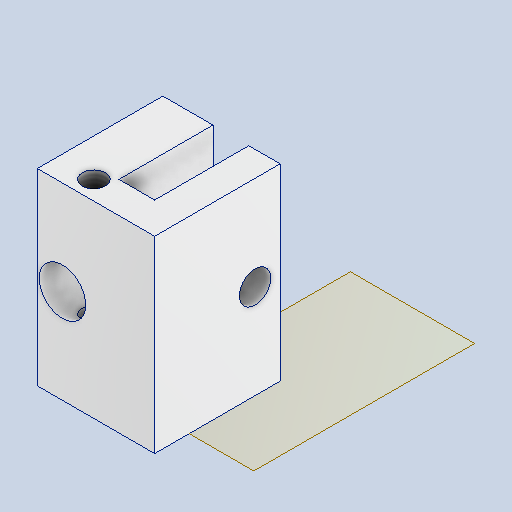
# Autodesk Inventor part: Katze_Lagerhalter_hinten
Saved by Autodesk Inventor 2025 (Build 290162010, 162A)
## iProperties
Created: 2024-11-11
Part Number: Katze_Lagerhalter_hinten
Material: Aluminium 6061(1)
Document SubType Name: Modeling
Designer: Admin
Density: 2.7 g/cm^3
Appearance: Aluminium - flach(1)
Author: Admin
Autodesk Inventor part; units mm, degrees
ref_plane "YZ Plane" through (0, 0, 0) normal (1, 0, 0) x (0, 1, 0)
ref_plane "XZ Plane" through (0, 0, 0) normal (0, 1, 0) x (-1, 0, 0)
ref_plane "XY Plane" through (0, 0, 0) normal (0, 0, 1) x (1, 0, 0)
ref_plane "Arbeitsebene1" through (0, 0, 0) normal (0, 0, 1) x (1, 0, 0)
sketch "Skizze1" plane through (0, 0, 0) normal (0, 0, 1) x (1, 0, 0)
  line L0 (-0.4, -3.1) -> (-5.4, -3.1)
  line L1 (-11.1, -3.1) -> (-19.1, -3.1)
  line L2 (-5.4, -3.1) -> (-5.4, -18.1)
  line L3 (-5.4, -18.1) -> (-11.1, -18.1)
  line L4 (-0.4, -23.1) -> (-0.4, -3.1)
  line L5 (-19.1, -23.1) -> (-0.4, -23.1)
  line L6 (-19.1, -3.1) -> (-19.1, -23.1)
  line L7 (-11.1, -18.1) -> (-11.1, -3.1)
  line L8 (-9, -16) -> (-9, -18.1) construction
  line L9 (-9, -16) -> (-11.1, -16) construction
  line L10 (-7.5, -16) -> (-5.4, -16) construction
  line L11 (-7.5, 1) -> (7.5, 1) projected
  line L12 (7.5, 1) -> (7.5, 16) projected
  line L13 (7.5, 16) -> (9, 16) projected
  line L14 (9, 16) -> (9, -16) projected
  line L15 (9, -16) -> (7.5, -16) projected
  line L16 (7.5, -16) -> (7.5, -1) projected
  line L17 (7.5, -1) -> (-7.5, -1) projected
  line L18 (-7.5, -1) -> (-7.5, -16) projected
  line L19 (-7.5, -16) -> (-9, -16) projected
  line L20 (-9, -16) -> (-9, 16) projected
  line L21 (-9, 16) -> (-7.5, 16) projected
  line L22 (-7.5, 16) -> (-7.5, 1) projected
  point P0 (0, 0)
  dimension "d0" = 5
  dimension "d1" = 8
  dimension "d2" = 5
  dimension "d3" = 20
  dimension "d4" = 2.1
  constraints: 22 end point, 10 perpendicular, 3 equal length, 3 point on line, 1 horizontal
  measures "d0" distance between parallel lines of L5 L3
  measures "d1" distance between parallel lines of L7 L6
  measures "d2" distance between parallel lines of L2 L4
  measures "d3" distance between parallel lines of L5 L1
  measures "d4" distance of L9.start L9.end
extrude "Extrusion1" add sketch "Skizze1" along normal blind 30 contours L4 L5 L6 L1 L7 L3 L2 L0
sketch "Skizze3" plane through (-5.4, -18.1, 0) normal (-1, 0, 0) x (0, 0, 1)
  line L0 (15, 6) -> (15, 15) construction
  line L1 (15, 6) -> (0, 6) construction
  line L2 (30, 15) -> (30, 0) construction
  line L3 (0, 15) -> (30, 15) construction
  line L4 (0, 15) -> (0, 0) construction
  line L5 (15, 6) -> (30, 6) construction
  point P0 (0, 18.1)
  dimension "d74" = 9
  constraints: 6 end point, 3 perpendicular, 2 point on line, 1 coincident, 1 collinear, 1 midpoint
  measures "d74" distance of L0.start L0.end
hole "GLHU" at (-5.4, -12.1, 15) direction (1, 0, 0) diameter 1.567 depth 4 tip angle 118 thread size "M2x0.4" class "6H" standard "ISO Metric profile"
sketch "Skizze9" plane through (-11.1, -18.1, 0) normal (0, 1, 0) x (1, 0, 0)
  line L0 (5.7, 0) -> (0, 0) construction
  line L1 (0, 0) -> (0, -30) construction
  line L2 (5.7, -30) -> (0, -30) construction
  line L3 (5.7, 0) -> (5.7, -30) construction
  line L4 (2.85, -30) -> (2.85, -15) construction
  line L5 (2.85, -15) -> (0, -15) construction
  line L6 (2.85, -15) -> (2.85, 0) construction
  point P0 (11.1, 0)
  constraints: 6 end point, 3 midpoint, 1 coincident, 1 collinear, 1 vertical
hole "GLHH" at (-8.25, -18.1, 15) direction (0, -1, 0) diameter 1.567 depth 4 tip angle 118 thread size "M2x0.4" class "6H" standard "ANSI Metric M Profile"
sketch "Skizze10" plane through (-11.1, -18.1, 0) normal (1, 0, 0) x (0, 0, -1)
  line L0 (-30, 0) -> (-30, 15) construction
  line L1 (0, 15) -> (-30, 15) construction
  line L2 (0, 0) -> (0, 15) construction
  line L3 (-30, 11) -> (-15, 11) construction
  line L4 (-15, 11) -> (0, 11) construction
  point P0 (0, 18.1)
  dimension "d75" = 4
  constraints: 4 end point, 3 point on line, 1 coincident, 1 collinear, 1 horizontal
  measures "d75" distance from line of L1 L3.end
hole "GLHO" at (-11.1, -7.1, 15) direction (-1, 0, 0) diameter 1.567 depth 4 tip angle 118 thread size "M2x0.4" class "6H" standard "ANSI Metric M Profile"
sketch "Skizze11" plane through (-11.1, -18.1, 0) normal (1, 0, 0) x (0, 0, -1)
  circle A0 centre (-15, 6) radius 0.7835 construction
  line L0 (0, 15) -> (0, 0) construction
  line L1 (0, 0) -> (-30, 0) construction
  line L2 (-30, 15) -> (-30, 0) construction
  line L3 (0, 15) -> (-30, 15) construction
  point P0 (0, 18.1)
  constraints: 1 coincident
hole "DLHO" at (-11.1, -12.1, 15) direction (-1, 0, 0) diameter 5 end through all
sketch "Skizze12" plane through (-5.4, -18.1, 0) normal (-1, 0, 0) x (0, 0, 1)
  circle A0 centre (15, 11) radius 0.7835 construction
  point P0 (0, 18.1)
  constraints: 1 coincident
hole "DLHU" at (-5.4, -7.1, 15) direction (1, 0, 0) diameter 5 end through all
sketch "Skizze6" plane through (-19.1, -3.1, 0) normal (0, 1, 0) x (1, 0, 0)
  line L0 (8, 0) -> (0, 0) projected
  line L1 (0, 0) -> (0, -30) projected
  line L2 (8, -30) -> (0, -30) projected
  line L3 (8, 0) -> (8, -30) projected
  line L4 (5.5, -30) -> (5.5, -27) construction
  line L5 (5.5, -27) -> (5.5, -3) construction
  line L6 (5.5, -3) -> (5.5, 0) construction
  line L7 (5.5, -3) -> (8, -3) construction
  point P0 (19.1, 0)
  dimension "d42" = 2.5
  dimension "d43" = 3
  constraints: 8 end point, 5 point on line, 2 coincident, 1 collinear, 1 perpendicular, 1 vertical
  measures "d42" distance of L5.end L7.end
  measures "d43" distance of L5.end L6.end
hole "Zentrierbolzen" at (-13.6, -3.1, 3) at (-13.6, -3.1, 27) direction (0, -1, 0) diameter 2 depth 5 tip angle 118
sketch "Skizze8" plane through (-19.1, -23.1, 0) normal (0, -1, 0) x (1, 0, 0)
  line L0 (0, 0) -> (18.7, 0) construction
  line L1 (18.7, 0) -> (18.7, 30) construction
  line L2 (0, 30) -> (18.7, 30) construction
  line L3 (0, 0) -> (0, 30) construction
  line L4 (4, 0) -> (4, 15) construction
  line L5 (4, 15) -> (4, 30) construction
  point P0 (19.1, 0)
  point P1 (0, 15)
  dimension "d58" = 4
  constraints: 4 end point, 3 point on line, 1 coincident, 1 collinear, 1 midpoint, 1 vertical
  measures "d58" distance of point (0, 15) L4.end
hole "LK-Verschraubung" at (-15.1, -23.1, 15) direction (0, 1, 0) diameter 4 end through all counterbore diameter 7.4 counterbore depth 14
sketch "Skizze13" plane through (0, 0, 0) normal (0, 0, -1) x (-1, 0, 0)
  line L0 (11.4, -9.1) -> (11.4, -23.1) construction
  line L1 (5.4, -18.1) -> (11.1, -18.1) construction
  line L2 (13.1, -20.1) -> (19.1, -20.1) construction
  line L3 (19.1, -3.1) -> (19.1, -23.1) construction
  line L4 (19.1, -23.1) -> (19.1, -20.1) construction
  point P0 (0, 0)
  dimension "d109" = 6
  dimension "d110" = 3
  constraints: 4 end point, 1 collinear, 1 horizontal, 1 point on line
  measures "d109" distance of L2.start L2.end
  measures "d110" distance of L3.end L2.end
hole "seiloese" at (-13.1, -20.1, 0) direction (0, 0, 1) diameter 3.6881 end through all thread size "M4.5x0.75" class "6H" standard "ANSI Metric M Profile"
thread "Gewinde4" size "M4x0.7" class "6H" standard "ANSI Metric M Profile" length 9
